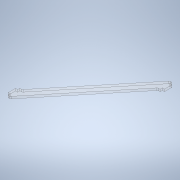
# Autodesk Inventor part: angularBrace
Saved by Autodesk Inventor 2020 (Build 240168000, 168)
## iProperties
Created: 2020-03-02
Part Number: angularBrace
Material: Polycarbonate, Clear
Document SubType Name: Modeling
Designer: n10208577
Density: 1.2 g/cm^3
Appearance: Polycarbonate - Clear
Author: n10208577
Autodesk Inventor part; units mm, degrees
ref_plane "YZ Plane" through (0, 0, 0) normal (1, 0, 0) x (0, 1, 0)
ref_plane "XZ Plane" through (0, 0, 0) normal (0, 1, 0) x (-1, 0, 0)
ref_plane "XY Plane" through (0, 0, 0) normal (0, 0, 1) x (1, 0, 0)
sketch "Sketch1" plane through (0, 0, 0) normal (0, 1, 0) x (-1, 0, 0)
  line L0 (-4.9492, -3.4256) -> (-7.9492, -3.4256)
  line L1 (-7.9492, -3.4256) -> (-7.9492, -13.4256)
  line L2 (-7.9492, -13.4256) -> (-4.9492, -13.4256)
  line L3 (-4.9492, -3.4256) -> (-4.9492, -0.4256)
  line L4 (-4.9492, -13.4256) -> (-4.9492, -16.4256)
  line L5 (-4.9492, -16.4256) -> (-2.8973, -16.4256)
  line L6 (-4.9492, -0.4256) -> (-2.8973, -0.4256)
  line L7 (91.2508, 106.8744) -> (94.2508, 106.8744)
  line L8 (94.2508, 106.8744) -> (94.2508, 96.8744)
  line L9 (94.2508, 96.8744) -> (91.2508, 96.8744)
  line L10 (91.2508, 106.8744) -> (91.2508, 109.8744)
  line L11 (91.2508, 96.8744) -> (91.2508, 93.8744)
  line L12 (91.2508, 93.8744) -> (89.1989, 93.8744)
  line L13 (91.2508, 109.8744) -> (89.1989, 109.8744)
  arc A0 (89.1989, 109.8744) -> (87.6506, 109.1404) centre (89.1989, 107.8744) ccw
  line L14 (-1.349, 0.3083) -> (87.6506, 109.1404)
  arc A1 (-2.8973, -0.4256) -> (-1.349, 0.3083) centre (-2.8973, 1.5744) ccw
  line L15 (-1.349, -15.6917) -> (87.6506, 93.1404)
  arc A2 (89.1989, 93.8744) -> (87.6506, 93.1404) centre (89.1989, 91.8744) ccw
  arc A3 (-2.8973, -16.4256) -> (-1.349, -15.6917) centre (-2.8973, -14.4256) ccw
  point P0 (0, 0)
  constraints: 32 end point, 8 point on circle, 4 centre point
extrude "Extrusion1" add sketch "Sketch1" along normal blind 3
body "Solid1"
